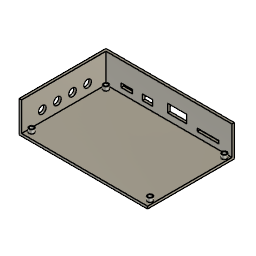
Untitledv1v2 (Autodesk Fusion 360 design; units mm, degrees)
part number: 2025-10-06-10-51-04-555
Autodesk Fusion 360 part; units mm, degrees
note: some values were not read from the file. Set by a fixed rule: which sketch regions a step uses.
sketch "Sketch1" plane through (0, 0, 0) normal (0, 0, 1) x (1, 0, 0)
  line L0 (0, 0) -> (100, 0)
  line L1 (100, 0) -> (100, -65)
  line L2 (100, -65) -> (0, -65)
  line L3 (0, -65) -> (0, 0)
  dimension "d1" = 100
  dimension "d2" = 65
  constraint horizontal L0
  constraint vertical L1
  constraint horizontal L2
  constraint vertical L3
  constraint coincident L0.start L3.end
  measures "d1" distance of L0.start L0.end
  measures "d2" distance of L0.start L2.end
extrude "Extrude1" add sketch "Sketch1" along normal blind 2
sketch "Sketch2" plane through (0, 0, 2) normal (0, 0, 1) x (-1, 0, 0)
  line L0 (0, 65) -> (-100, 65)
  line L1 (-100, 65) -> (-100, 0)
  line L2 (-100, 0) -> (0, 0)
  line L3 (0, 0) -> (0, 65)
  line L4 (0, 65) -> (-120, 65)
  line L5 (-120, 65) -> (-210, 65)
  line L6 (-210, 65) -> (-290, 65)
  line L7 (-290, 65) -> (-370, 65)
  line L8 (-370, 65) -> (-490, 65)
  line L9 (-490, 65) -> (-640, 65)
  line L10 (-640, 65) -> (-725, 65)
  line L11 (-725, 65) -> (-895, 65)
  line L12 (-895, 65) -> (-1000, 65)
  line L13 (0, 0) -> (-1.5, 0)
  line L14 (-1.5, 0) -> (-1.5, 1.5)
  line L15 (-1.5, 1.5) -> (-1.5, 3)
  line L16 (-1.5, 3) -> (-3, 3)
  circle A0 centre (-3, 3) radius 1.5
  circle A1 centre (-3, 3) radius 2
  dimension "d5" = 120
  dimension "d6" = 90
  dimension "d7" = 80
  dimension "d8" = 80
  dimension "d9" = 120
  dimension "d10" = 150
  dimension "d11" = 85
  dimension "d12" = 170
  dimension "d13" = 105
  dimension "d14" = 1.5
  dimension "d15" = 1.5
  dimension "d16" = 1.5
  dimension "d17" = 1.5
  dimension "d18" = 3
  constraint coincident L0.start L3.end
  constraint perpendicular L3 L4
  constraint parallel L0 L5
  constraint parallel L0 L6
  constraint parallel L0 L7
  constraint parallel L0 L8
  constraint parallel L0 L9
  constraint parallel L0 L10
  constraint parallel L0 L11
  constraint perpendicular L1 L12
  constraint coincident L2.end L3.start
  constraint perpendicular L3 L13
  constraint perpendicular L13 L14
  constraint parallel L14 L15
  constraint perpendicular L15 L16
  constraint coincident L16.end A0.centre
  measures "d5" distance of L0.start L4.end
  measures "d6" distance of L4.end L5.end
  measures "d7" distance of L5.end L6.end
  measures "d8" distance of L6.end L7.end
  measures "d9" distance of L7.end L8.end
  measures "d10" distance of L8.end L9.end
  measures "d11" distance of L9.end L10.end
  measures "d12" distance of L10.end L11.end
  measures "d13" distance of L11.end L12.end
  measures "d14" distance of L2.end L13.end
  measures "d15" distance of L13.end L14.end
  measures "d16" distance of L14.end L15.end
  measures "d17" distance of L15.end L16.end
  measures "d18" diameter of A0
extrude "Extrude2" add sketch "Sketch2" along normal blind 3 contours A1
pattern_linear "R-Pattern2" count 2 spacing 94 along (1, 0, 0) count 2 spacing 59 along (0, -1, 0) of "Extrude2"
sketch "Sketch4" plane through (0, 0, 0) normal (0, 0, -1) x (1, 0, 0)
  line L0 (100, 65) -> (0, 65)
  line L1 (0, 65) -> (0, 0)
  line L2 (0, 0) -> (100, 0)
  line L3 (100, 0) -> (100, 65)
  line L4 (0, 0) -> (-2, 0)
  line L5 (-2, 0) -> (-2, 65)
  line L6 (-2, 65) -> (0, 65)
  line L7 (0, 65) -> (0, 0)
  line L8 (-2, 65) -> (100, 65)
  line L9 (100, 65) -> (100, 67)
  line L10 (100, 67) -> (-2, 67)
  line L11 (-2, 67) -> (-2, 65)
  dimension "d37" = 2
  dimension "d38" = 2
  constraint horizontal L4
  constraint vertical L5
  constraint horizontal L6
  constraint vertical L7
  constraint coincident L1.end L2.start
  constraint horizontal L8
  constraint vertical L9
  constraint horizontal L10
  constraint vertical L11
  measures "d37" distance of L1.end L4.end
  measures "d38" distance of L5.end L10.end
extrude "Extrude6" add sketch "Sketch4" against normal blind 25 contours L0 L6 L8 L9 L10 L11 | L1 L4 L5 L6 L7 L8
sketch "Sketch5" plane through (0, -67, 0) normal (0, -1, 0) x (1, 0, 0)
  line L0 (-2, 0) -> (100, 0)
  line L1 (100, 0) -> (100, 25)
  line L2 (100, 25) -> (-2, 25)
  line L3 (-2, 25) -> (-2, 0)
  line L4 (0, 25) -> (0, 0) construction
  line L5 (0, 5) -> (100, 5) construction
  line L6 (0, 5) -> (100, 5)
  line L7 (100, 5) -> (100, 6.15)
  line L8 (100, 6.15) -> (0, 6.15)
  line L9 (0, 6.15) -> (0, 5)
  line L10 (0, 6.15) -> (12, 6.15)
  line L11 (12, 6.15) -> (21, 6.15)
  line L12 (21, 6.15) -> (21, 9.15)
  line L13 (21, 9.15) -> (12, 9.15)
  line L14 (12, 9.15) -> (12, 6.15)
  line L15 (21, 6.15) -> (29, 6.15)
  line L16 (29, 6.15) -> (37, 6.15)
  line L17 (37, 6.15) -> (37, 10.15)
  line L18 (37, 10.15) -> (29, 10.15)
  line L19 (29, 10.15) -> (29, 6.15)
  line L20 (37, 6.15) -> (49, 6.15)
  line L21 (49, 6.15) -> (64, 6.15)
  line L22 (64, 6.15) -> (64, 13.65)
  line L23 (64, 13.65) -> (49, 13.65)
  line L24 (49, 13.65) -> (49, 6.15)
  line L25 (64, 6.15) -> (72.5, 6.15)
  line L26 (72.5, 6.15) -> (89.5, 6.15)
  line L27 (89.5, 6.15) -> (89.5, 8.35)
  line L28 (89.5, 8.35) -> (72.5, 8.35)
  line L29 (72.5, 8.35) -> (72.5, 6.15)
  line L30 (89.5, 6.15) -> (100, 6.15)
  line L31 (49, 6.15) -> (49, 7.15)
  line L32 (49, 7.15) -> (64, 7.15)
  line L33 (29, 6.15) -> (29, 5.65)
  line L34 (29, 5.65) -> (37, 5.65)
  line L35 (37, 5.65) -> (37, 6.15)
  dimension "d41" = 1.15
  dimension "d42" = 12
  dimension "d43" = 9
  dimension "d44" = 3
  dimension "d45" = 8
  dimension "d46" = 8
  dimension "d47" = 4
  dimension "d48" = 12
  dimension "d49" = 15
  dimension "d50" = 7.5
  dimension "d51" = 8.5
  dimension "d52" = 17
  dimension "d53" = 2.2
  dimension "d73" = 1
  dimension "d74" = 0.5
  constraint coincident L2 L4.start
  constraint coincident L4.end origin
  constraint perpendicular L0 L4
  constraint coincident L4 L5.start
  constraint coincident L1 L5.end
  constraint perpendicular L1 L5
  constraint horizontal L6
  constraint vertical L7
  constraint horizontal L8
  constraint vertical L9
  constraint coincident L1 L7.end
  constraint perpendicular L9 L10
  constraint horizontal L11
  constraint vertical L12
  constraint horizontal L13
  constraint vertical L14
  constraint perpendicular L12 L15
  constraint horizontal L16
  constraint vertical L17
  constraint horizontal L18
  constraint vertical L19
  constraint perpendicular L17 L20
  constraint horizontal L21
  constraint vertical L22
  constraint horizontal L23
  constraint vertical L24
  constraint perpendicular L22 L25
  constraint horizontal L26
  constraint vertical L27
  constraint horizontal L28
  constraint vertical L29
  constraint perpendicular L20 L31
  constraint coincident L22 L32.end
  constraint perpendicular L22 L32
  constraint perpendicular L16 L33
  constraint perpendicular L33 L34
  measures "d41" distance of L5.start L8.end
  measures "d42" distance of L8.end L10.end
  measures "d43" distance of L10.end L11.end
  measures "d44" distance of L10.end L13.end
  measures "d45" distance of L11.end L15.end
  measures "d46" distance of L15.end L16.end
  measures "d47" distance of L15.end L18.end
  measures "d48" distance of L16.end L20.end
  measures "d49" distance of L20.end L21.end
  measures "d50" distance of L20.end L23.end
  measures "d51" distance of L21.end L25.end
  measures "d52" distance of L25.end L26.end
  measures "d53" distance of L25.end L28.end
  measures "d73" distance of L20.end L31.end
  measures "d74" distance of L15.end L33.end
extrude "Extrude7" cut sketch "Sketch5" against normal up to surface (2 mm away) contours L8 L26 L27 L28 L29 | L8 L11 L12 L13 L14 | L22 L23 L24 L32 | L8 L16 L17 L18 L19 | L8 L16 L33 L34 L35
sketch "Sketch6" plane through (-2, 0, 0) normal (-1, 0, 0) x (0, -1, 0)
  line L0 (0, 0) -> (67, 0)
  line L1 (67, 0) -> (67, 25)
  line L2 (67, 25) -> (0, 25)
  line L3 (0, 25) -> (0, 0)
  line L4 (65, 25) -> (65, 0)
  line L5 (67, 5) -> (0, 5)
  line L6 (67, 5) -> (0, 5)
  line L7 (0, 5) -> (0, 6.15)
  line L8 (0, 6.15) -> (67, 6.15) construction
  line L9 (67, 6.15) -> (67, 5)
  line L10 (65, 5) -> (65, 10)
  line L11 (65, 10) -> (0, 10)
  line L12 (65, 10) -> (50.5, 10)
  circle A0 centre (50.5, 10) radius 3
  line L13 (50.5, 10) -> (38.5, 10)
  circle A1 centre (38.5, 10) radius 3
  line L14 (38.5, 10) -> (26.5, 10)
  circle A2 centre (26.5, 10) radius 3
  line L15 (26.5, 10) -> (14.5, 10)
  circle A3 centre (14.5, 10) radius 3
  dimension "d56" = 67
  dimension "d57" = 1.15
  dimension "d58" = 5
  dimension "d59" = 14.5
  dimension "d60" = 6
  dimension "d61" = 12
  dimension "d62" = 12
  dimension "d63" = 12
  constraint coincident L2 L4.start
  constraint coincident L0 L4.end
  constraint perpendicular L0 L4
  constraint coincident L1 L5.start
  constraint coincident L3 L5.end
  constraint perpendicular L3 L5
  constraint horizontal L6
  constraint vertical L7
  constraint horizontal L8
  constraint vertical L9
  constraint coincident L6 L10.start
  constraint coincident L4 L10.start
  constraint perpendicular L5 L10
  constraint coincident L3 L11.end
  constraint perpendicular L3 L11
  constraint perpendicular L10 L12
  constraint coincident L12.end A0.centre
  constraint parallel L11 L13
  constraint coincident L13.end A1.centre
  constraint parallel L11 L14
  constraint coincident L14.end A2.centre
  constraint parallel L11 L15
  constraint coincident L15.end A3.centre
  measures "d56" distance of L5.start L5.end
  measures "d57" distance of L5.start L8.end
  measures "d58" distance of L10.start L10.end
  measures "d59" distance of L10.end L12.end
  measures "d60" diameter of A0
  measures "d61" distance of L12.end L13.end
  measures "d62" distance of L13.end L14.end
  measures "d63" distance of L14.end L15.end
ref_plane "WorkPlane1" through (50, -32.5, 13.5) normal (0, 1, 0) x (-1, 0, 0)
mirror "Mirror1" about plane through (50, -32.5, 13.5) normal (0, 1, 0) of "Extrude6"
extrude "Extrude8" cut sketch "Sketch6" against normal up to surface (2 mm away) contours L11 L12 A0 L13 | L11 L12 A0 L13 | L11 L15 A3 | L11 L15 A3 | L11 L13 A1 L14 | L11 L13 A1 L14 | L11 L14 A2 L15 | L11 L14 A2 L15
mirror "Mirror2" about plane through (50, -32.5, 13.5) normal (0, 1, 0) of "Extrude7"
sketch "Sketch7" plane through (0, 0, 25) normal (0, 0, 1) x (-1, 0, 0)
  line L0 (2, -2) -> (2, 67)
  line L1 (2, 67) -> (-100, 67)
  line L2 (-100, 67) -> (-100, 65)
  line L3 (-100, 65) -> (0, 65)
  line L4 (0, 65) -> (0, 0)
  line L5 (0, 0) -> (-100, 0)
  line L6 (-100, 0) -> (-100, -2)
  line L7 (-100, -2) -> (2, -2)
  line L8 (0, 65) -> (-100, 65)
  line L9 (-100, 65) -> (-100, 67)
  line L10 (-100, 67) -> (0, 67)
  line L11 (0, 67) -> (0, 65)
  constraint horizontal L8
  constraint vertical L9
  constraint horizontal L10
  constraint vertical L11
  constraint coincident L1.end L2.start
  constraint coincident L3.end L4.start
extrude "Extrude9" cut sketch "Sketch7" against normal blind 23 contours L1 L2 L3 L8 L9 L10 L11
